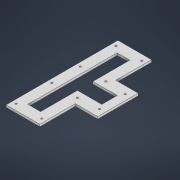
# Autodesk Inventor part: Diff_test_2
Saved by Autodesk Inventor 2021 (Build 250183000, 183)
## iProperties
Created: 2021-03-03
Part Number: Diff_test_2
Material: Generisch
Document SubType Name: Modeling
Designer: Ctroi
Density: 1 g/cm^3
Appearance: Vorgabe
Author: Ctroi
## iProperties of the stored document _3D-Druck.ipt
Created: 2021-03-03
Part Number: _3D-Druck
Material: Generisch
Document SubType Name: Modeling
Designer: Ctroi
Density: 1 g/cm^3
Appearance: Vorgabe
Author: Ctroi
Autodesk Inventor part; units mm, degrees
ref_plane "YZ Plane" through (0, 0, 0) normal (1, 0, 0) x (0, 1, 0)
ref_plane "XZ Plane" through (0, 0, 0) normal (0, 1, 0) x (-1, 0, 0)
ref_plane "XY Plane" through (0, 0, 0) normal (0, 0, 1) x (1, 0, 0)
sketch "Skizze1" plane through (0, 0, 0) normal (0, 1, 0) x (-1, 0, 0)
  line L0 (-30, 100) -> (30, 100)
  line L1 (30, 100) -> (30, -100)
  line L2 (30, -100) -> (-30, -100)
  line L3 (-30, -100) -> (-30, 100)
  line L4 (-30, 100) -> (30, -100) construction
  line L5 (30, 100) -> (-30, -100) construction
  line L6 (0, -140) -> (0, 140) projected
  line L7 (-42, 0) -> (42, 0) projected
  point P0 (0, 0)
  point P1 (0, 0)
  dimension "d0" = 60
  dimension "d1" = 200
  constraints: 12 end point, 2 midpoint, 2 parallel, 1 horizontal, 1 perpendicular, 2 other
  measures "d0" distance between parallel lines of L1 L3
  measures "d1" distance between parallel lines of L0 L2
extrude "Extrusion1" add sketch "Skizze1" along normal blind 2
sketch "Skizze3" plane through (30, 0, 100) normal (1, 0, 0) x (0, 0, -1)
  line L0 (200, 2) -> (0, 2) projected
  line L1 (200, 0) -> (0, 0) projected
  line L2 (63.8142, 2) -> (136.1858, 2)
  line L3 (136.1858, 2) -> (136.1858, 0)
  line L4 (136.1858, 0) -> (63.8142, 0)
  line L5 (63.8142, 0) -> (63.8142, 2)
  line L6 (100, -0.4) -> (100, 2.4) projected
  point P0 (100, 0)
  constraints: 8 end point, 2 parallel, 2 point on line, 1 horizontal, 1 perpendicular, 1 other
extrude "Extrusion3" add sketch "Skizze3" along normal blind 40
sketch "Skizze2" plane through (0, 2, 0) normal (0, 1, 0) x (1, 0, 0)
  line L0 (0, 140) -> (0, -140) projected
  line L1 (90, 0) -> (-50, 0) projected
  circle A0 centre (-23, 89.5) radius 1.6
  circle A1 centre (23, 89.5) radius 1.6
  line L2 (30, 100) -> (-30, 100) projected
  circle A2 centre (-23, 25.5) radius 1.6
  circle A3 centre (23, 25.5) radius 1.6
  circle A4 centre (-23, -89.5) radius 1.6
  circle A5 centre (23, -89.5) radius 1.6
  circle A6 centre (-23, -25.5) radius 1.6
  circle A7 centre (23, -25.5) radius 1.6
  line L3 (25, 83.9) -> (25, 31.1)
  line L4 (-25, 31.1) -> (-25, 83.9)
  line L5 (-30, 100) -> (-30, -100) projected
  line L6 (30, -100) -> (30, 100) projected
  line L7 (-17.4, 96) -> (17.4, 96)
  line L8 (17.4, 96) -> (17.4, 83.9)
  line L9 (-17.4, 83.9) -> (-17.4, 96)
  line L10 (-25, 83.9) -> (-17.4, 83.9)
  line L11 (17.4, 83.9) -> (25, 83.9)
  line L12 (17.4, -96) -> (-17.4, -96)
  line L13 (25, 31.1) -> (17.4, 31.1)
  line L14 (-17.4, 31.1) -> (-25, 31.1)
  line L15 (-30, -100) -> (30, -100) projected
  line L16 (-17.4, -31.1) -> (-26, -31.1)
  line L17 (-26, -31.1) -> (-26, -83.9)
  line L18 (-26, -83.9) -> (-17.4, -83.9)
  line L19 (17.4, -31.1) -> (26, -31.1)
  line L20 (26, -31.1) -> (26, -83.9)
  line L21 (26, -83.9) -> (17.4, -83.9)
  line L22 (-17.4, 19.9) -> (-26, 19.9)
  line L23 (-26, 19.9) -> (-26, -19.9)
  line L24 (-26, -19.9) -> (-17.4, -19.9)
  line L25 (17.4, 19.9) -> (26, 19.9)
  line L26 (26, 19.9) -> (26, -19.9)
  line L27 (26, -19.9) -> (17.4, -19.9)
  line L28 (-17.4, 19.9) -> (-17.4, 31.1)
  line L29 (17.4, 31.1) -> (17.4, 19.9)
  line L30 (17.4, -19.9) -> (17.4, -31.1)
  line L31 (17.4, -83.9) -> (17.4, -96)
  line L32 (-17.4, -96) -> (-17.4, -83.9)
  line L33 (-17.4, -31.1) -> (-17.4, -19.9)
  circle A8 centre (60, 23) radius 1.6
  circle A9 centre (60, -23) radius 1.6
  line L34 (30, 32.1858) -> (54.4, 32.1858)
  line L35 (54.4, -32.1858) -> (30, -32.1858)
  line L36 (30, -32.1858) -> (30, 32.1858)
  line L37 (30, -36.1858) -> (70, -36.1858) projected
  line L38 (30, 36.1858) -> (70, 36.1858) projected
  line L39 (54.4, 17.4) -> (66, 17.4)
  line L40 (66, 17.4) -> (66, -17.4)
  line L41 (66, -17.4) -> (54.4, -17.4)
  line L42 (70, 36.1858) -> (70, -36.1858) projected
  line L43 (54.4, 32.1858) -> (66, 32.1858)
  line L44 (66, 32.1858) -> (66, 28.6)
  line L45 (66, 28.6) -> (54.4, 28.6)
  line L46 (54.4, -28.6) -> (66, -28.6)
  line L47 (66, -28.6) -> (66, -32.1858)
  line L48 (66, -32.1858) -> (54.4, -32.1858)
  line L49 (54.4, 28.6) -> (54.4, 17.4)
  line L50 (54.4, -17.4) -> (54.4, -28.6)
  point P0 (0, 0)
  dimension "d2" = 2
  dimension "d4" = 3.2
  dimension "d5" = 3.2
  dimension "d6" = 10.5
  dimension "d7" = 10.5
  dimension "d8" = 23
  dimension "d9" = 23
  dimension "d10" = 3.2
  dimension "d11" = 3.2
  dimension "d12" = 23
  dimension "d13" = 23
  dimension "d14" = 25.5
  dimension "d15" = 25.5
  dimension "d16" = 5
  dimension "d17" = 5
  dimension "d23" = 4
  dimension "d24" = 4
  dimension "d25" = 4
  dimension "d26" = 4
  dimension "d27" = 4
  dimension "d30" = 4
  dimension "d31" = 4
  dimension "d33" = 4
  dimension "d34" = 4
  dimension "d35" = 4
  dimension "d36" = 4
  dimension "d37" = 4
  dimension "d38" = 4
  dimension "d39" = 4
  dimension "d40" = 4
  dimension "d41" = 4
  dimension "d42" = 4
  dimension "d43" = 4
  dimension "d44" = 4
  dimension "d45" = 4
  dimension "d48" = 12.6
  dimension "d49" = 12.6
  dimension "d50" = 12.6
  dimension "d51" = 12.6
  dimension "d52" = 12.6
  dimension "d53" = 12.6
  dimension "d58" = 3.2
  dimension "d59" = 3.2
  dimension "d60" = 23
  dimension "d61" = 23
  dimension "d64" = 37
  dimension "d65" = 37
  dimension "d66" = 4
  dimension "d68" = 4
  dimension "d69" = 4
  dimension "d70" = 4
  dimension "d71" = 4
  dimension "d72" = 4
  dimension "d73" = 4
  dimension "d74" = 4
  dimension "d75" = 4
  dimension "d76" = 4
  dimension "d77" = 15.6
  dimension "d78" = 15.6
  constraints: 84 end point, 25 parallel, 12 perpendicular, 11 horizontal, 10 centre point, 4 symmetric about line, 1 point on line, 4 other
  measures "d4" diameter of A0
  measures "d5" diameter of A1
  measures "d6" distance from line of L2 A0.centre
  measures "d7" distance from line of L2 A1.centre
  measures "d8" distance from line of L0 A0.centre
  measures "d9" distance from line of L0 A1.centre
  measures "d10" diameter of A2
  measures "d11" diameter of A3
  measures "d12" distance from line of L0 A2.centre
  measures "d13" distance from line of L0 A3.centre
  measures "d14" distance from line of L1 A2.centre
  measures "d15" distance from line of L1 A3.centre
  measures "d16" distance between parallel lines of L5 L4
  measures "d17" distance between parallel lines of L6 L3
  measures "d23" distance edge to line of A1 L11
  measures "d24" distance edge to line of A0 L10
  measures "d25" distance between parallel lines of L2 L7
  measures "d26" distance edge to line of A1 L8
  measures "d27" distance edge to line of A0 L9
  measures "d30" distance edge to line of A3 L13
  measures "d31" distance edge to line of A2 L14
  measures "d33" distance between parallel lines of L15 L12
  measures "d34" distance edge to line of A6 L16
  measures "d35" distance between parallel lines of L5 L17
  measures "d36" distance edge to line of A4 L18
  measures "d37" distance edge to line of A7 L19
  measures "d38" distance edge to line of A5 L21
  measures "d39" distance between parallel lines of L6 L20
  measures "d40" distance edge to line of A2 L22
  measures "d41" distance between parallel lines of L5 L23
  measures "d42" distance edge to line of A6 L24
  measures "d43" distance between parallel lines of L6 L26
  measures "d44" distance edge to line of A3 L25
  measures "d45" distance edge to line of A7 L27
  measures "d48" distance between parallel lines of L5 L28
  measures "d49" distance between parallel lines of L6 L29
  measures "d50" distance between parallel lines of L6 L30
  measures "d51" distance between parallel lines of L5 L33
  measures "d52" distance between parallel lines of L5 L32
  measures "d53" distance between parallel lines of L6 L31
  measures "d58" diameter of A8
  measures "d59" diameter of A9
  measures "d60" distance from line of L1 A8.centre
  measures "d61" distance from line of L1 A9.centre
  measures "d64" horizontal distance of A3.centre A8.centre
  measures "d65" horizontal distance of A7.centre A9.centre
  measures "d66" distance between parallel lines of L37 L35
  measures "d68" distance between parallel lines of L38 L34
  measures "d69" distance edge to line of A8 L39
  measures "d70" distance edge to line of A9 L41
  measures "d71" distance between parallel lines of L42 L40
  measures "d72" distance edge to line of A8 L45
  measures "d73" distance between parallel lines of L42 L44
  measures "d74" distance edge to line of A9 L46
  measures "d75" distance between parallel lines of L37 L48
  measures "d76" distance between parallel lines of L42 L47
  measures "d77" distance between parallel lines of L42 L49
  measures "d78" distance between parallel lines of L42 L50
extrude "Extrusion2" cut sketch "Skizze2" against normal up to surface (2 mm away) contours A0 | A1 | A2 | A3 | A4 | A5 | A6 | A7 | A8 | A9
sketch "Skizze4" plane through (0, 0, 0) normal (0, -1, 0) x (1, 0, 0)
  circle A0 centre (-23, -89.5) radius 1.6 projected
  circle A1 centre (60, -23) radius 1.6 projected
  circle A2 centre (23, -25.5) radius 1.6 projected
  circle A3 centre (-23, 89.5) radius 1.6 projected
  circle A4 centre (23, 25.5) radius 1.6 projected
  circle A5 centre (23, -89.5) radius 1.6 projected
  circle A6 centre (60, 23) radius 1.6 projected
  circle A7 centre (-23, -25.5) radius 1.6 projected
  circle A8 centre (23, 89.5) radius 1.6 projected
  circle A9 centre (-23, 25.5) radius 1.6 projected
  line L0 (-30, -100) -> (-30, 100) projected
  line L1 (30, -100) -> (-30, -100) projected
  line L2 (30, -36.1858) -> (30, -100) projected
  line L3 (30, -36.1858) -> (70, -36.1858) projected
  line L4 (70, 36.1858) -> (70, -36.1858) projected
  line L5 (30, 36.1858) -> (70, 36.1858) projected
  line L6 (30, 100) -> (30, 36.1858) projected
  line L7 (-30, 100) -> (30, 100) projected
  point P0 (0, 0)
extrude "Extrusion4" add sketch "Skizze4" along normal blind 2
sketch "Skizze5" plane through (0, 2, 0) normal (0, 1, 0) x (1, 0, 0)
  line L0 (-11.4, 79.9) -> (11.4, 79.9)
  line L1 (11.4, -79.9) -> (-11.4, -79.9)
  line L2 (-11.4, -79.9) -> (-11.4, 79.9)
  circle A0 centre (-23, 25.5) radius 1.6 projected
  circle A1 centre (23, 25.5) radius 1.6 projected
  circle A2 centre (23, 89.5) radius 1.6 projected
  circle A3 centre (-23, -89.5) radius 1.6 projected
  line L3 (11.4, 13.9) -> (55, 13.9)
  line L4 (55, 13.9) -> (55, -13.9)
  line L5 (55, -13.9) -> (11.4, -13.9)
  line L6 (70, 36.1858) -> (70, -36.1858) projected
  circle A4 centre (23, -25.5) radius 1.6 projected
  line L7 (11.4, 79.9) -> (11.4, 13.9)
  line L8 (11.4, -13.9) -> (11.4, -79.9)
  line L9 (30, 36.1858) -> (30, 100) projected
  line L10 (30, -100) -> (30, -36.1858) projected
  point P0 (0, 0)
  dimension "d81" = 10
  dimension "d83" = 8
  dimension "d84" = 8
  dimension "d85" = 15
  dimension "d86" = 10
  dimension "d87" = 10
  dimension "d88" = 18.6
  dimension "d89" = 18.6
  constraints: 16 end point, 4 parallel, 3 perpendicular, 2 horizontal
  measures "d81" distance edge to line of A0 L2
  measures "d83" distance edge to line of A2 L0
  measures "d84" distance edge to line of A3 L1
  measures "d85" distance between parallel lines of L6 L4
  measures "d86" distance edge to line of A1 L3
  measures "d87" distance edge to line of A4 L5
  measures "d88" distance between parallel lines of L9 L7
  measures "d89" distance between parallel lines of L10 L8
extrude "Extrusion5" cut sketch "Skizze5" against normal up to surface (4 mm away) contours L0 L7 L3 L4 L5 L8 L1 L2
